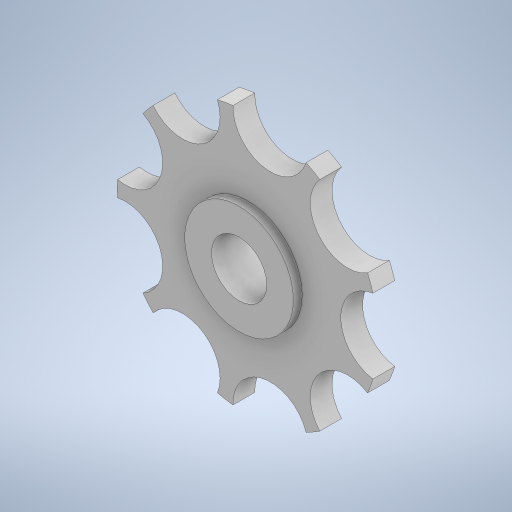
# Autodesk Inventor part: Gear
Saved by Autodesk Inventor 2024 (Build 280153000, 153)
## iProperties
Created: 2024-02-05
Part Number: Gear
Material: Generic
Document SubType Name: Modeling
Designer: Ramji Yadav
Density: 1 g/cm^3
Appearance: Default
Author: Ramji Yadav
Autodesk Inventor part; units mm, degrees
ref_plane "YZ Plane" through (0, 0, 0) normal (1, 0, 0) x (0, 1, 0)
ref_plane "XZ Plane" through (0, 0, 0) normal (0, 1, 0) x (-1, 0, 0)
ref_plane "XY Plane" through (0, 0, 0) normal (0, 0, 1) x (1, 0, 0)
sketch "Sketch1" plane through (0, 0, 0) normal (0, 0, 1) x (1, 0, 0)
  circle A0 centre (0, 0) radius 6.35
  circle A1 centre (0, 0) radius 21.3337
  arc A2 (28.7594, 8.538) -> (28.7594, -8.538) centre (30, 0) ccw
  arc A3 (16.5428, 25.0267) -> (27.5191, 11.9457) centre (22.9813, 19.2836) ccw
  arc A4 (-3.4143, 29.8051) -> (13.4023, 26.8399) centre (5.2094, 29.5442) ccw
  arc A5 (-21.7738, 20.6373) -> (-6.9856, 29.1754) centre (-15, 25.9808) ccw
  arc A6 (-29.9452, 1.8132) -> (-24.1048, 17.8594) centre (-28.1908, 10.2606) ccw
  arc A7 (-24.1048, -17.8594) -> (-29.9452, -1.8132) centre (-28.1908, -10.2606) ccw
  arc A8 (-6.9856, -29.1754) -> (-21.7738, -20.6373) centre (-15, -25.9808) ccw
  arc A9 (13.4023, -26.8399) -> (-3.4143, -29.8051) centre (5.2094, -29.5442) ccw
  arc A10 (27.5191, -11.9457) -> (16.5428, -25.0267) centre (22.9813, -19.2836) ccw
  arc A11 (27.5191, -11.9457) -> (28.7594, -8.538) centre (0, 0) ccw
  arc A12 (28.7594, 8.538) -> (27.5191, 11.9457) centre (0, 0) ccw
  arc A13 (16.5428, 25.0267) -> (13.4023, 26.8399) centre (0, 0) ccw
  arc A14 (-3.4143, 29.8051) -> (-6.9856, 29.1754) centre (0, 0) ccw
  arc A15 (-21.7738, 20.6373) -> (-24.1048, 17.8594) centre (0, 0) ccw
  arc A16 (-29.9452, 1.8132) -> (-29.9452, -1.8132) centre (0, 0) ccw
  arc A17 (-24.1048, -17.8594) -> (-21.7738, -20.6373) centre (0, 0) ccw
  arc A18 (-6.9856, -29.1754) -> (-3.4143, -29.8051) centre (0, 0) ccw
  arc A19 (13.4023, -26.8399) -> (16.5428, -25.0267) centre (0, 0) ccw
  arc A20 (-6.3913, -25.4085) -> (-2.6843, -26.0621) centre (0, 0) ccw
  point P0 (25.2001, -7.1692)
  point P1 (25.2001, 7.1692)
  point P2 (23.9126, 10.7064)
  point P3 (14.6961, 21.6902)
  point P4 (11.4362, 23.5723)
  point P5 (-2.6843, 26.0621)
  point P6 (-6.3913, 25.4085)
  point P7 (-18.8087, 18.2393)
  point P8 (-21.2283, 15.3558)
  point P9 (-26.1323, 1.8821)
  point P10 (-26.1323, -1.8821)
  point P11 (-21.2283, -15.3558)
  point P12 (-18.8087, -18.2393)
  point P13 (11.4362, -23.5723)
  point P14 (23.9126, -10.7064)
  point P15 (14.6961, -21.6902)
  dimension "d1" = 12.7
  dimension "d5" = 360
  constraints: 56 point on circle, 21 centre point, 6 coincident, 62 other
  measures "d1" diameter of A0
extrude "Extrusion1" add sketch "Sketch1" along normal blind 5 contours A0 | A1 | A2 A11 A10 A19 A9 A20 A8 A17 A7 A16 A6 A15 A5 A14 A4 A13 A3 A12 | A9 A18 A8 A20
sketch "Sketch2" plane through (0, 0, 5) normal (0, 0, 1) x (1, 0, 0)
  circle A0 centre (0, 0) radius 6.35
  dimension "d9" = 12.7
  constraints: 1 centre point, 1 coincident
  measures "d9" diameter of A0
extrude "Extrusion2" cut sketch "Sketch2" against normal through all
sketch "Sketch3" plane through (0, 0, 5) normal (0, 0, 1) x (1, 0, 0)
  circle A0 centre (0, 0) radius 12.5
  circle A1 centre (0, 0) radius 6.35
  dimension "d12" = 25
  dimension "d13" = 12.7
  constraints: 2 centre point, 2 coincident
  measures "d12" diameter of A0
  measures "d13" diameter of A1
extrude "Extrusion3" add sketch "Sketch3" along normal blind 2
sketch "Sketch4" plane through (0, 0, 0) normal (0, 0, -1) x (-1, 0, 0)
  circle A0 centre (0, 0) radius 6.35
  circle A1 centre (0, 0) radius 12.5
  dimension "d16" = 12.7
  dimension "d17" = 25
  constraints: 2 centre point, 2 coincident
  measures "d16" diameter of A0
  measures "d17" diameter of A1
extrude "Extrusion4" add sketch "Sketch4" along normal blind 2
body "Solid1"
